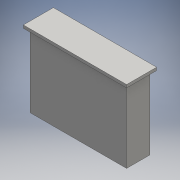
# Autodesk Inventor part: 240531_3Dstorage2
Saved by Autodesk Inventor 2016 (Build 200138000, 138)
## iProperties
Created: 2024-05-31
Part Number: 240531_3Dstorage2
Material: 일반
Document SubType Name: Modeling
Designer: pc
Density: 1 g/cm^3
Appearance: 기본값
Author: pc
Autodesk Inventor part; units mm, degrees
ref_plane "YZ Plane" through (0, 0, 0) normal (1, 0, 0) x (0, 1, 0)
ref_plane "XZ Plane" through (0, 0, 0) normal (0, 1, 0) x (-1, 0, 0)
ref_plane "XY Plane" through (0, 0, 0) normal (0, 0, 1) x (1, 0, 0)
sketch "스케치1" plane through (0, 0, 0) normal (0, 0, 1) x (1, 0, 0)
  line L0 (250, -60) -> (-250, -60)
  line L1 (-250, -60) -> (-250, 60)
  line L2 (-250, 60) -> (250, 60)
  line L3 (250, 60) -> (250, -60)
  line L4 (250, -60) -> (-250, 60) construction
  line L5 (-250, -60) -> (250, 60) construction
  point P0 (0, 0)
  dimension "d0" = 500
  dimension "d1" = 120
  constraints: 12 end point, 2 midpoint, 2 parallel, 1 horizontal, 1 perpendicular
  measures "d0" distance of L1.end L2.end
  measures "d1" distance of L2.end L0.start
extrude "돌출1" add sketch "스케치1" along normal blind 380
sketch "스케치2" plane through (0, 0, 380) normal (0, 0, 1) x (1, 0, 0)
  line L0 (-268, 78) -> (268, 78)
  line L1 (268, 78) -> (268, -78)
  line L2 (268, -78) -> (-268, -78)
  line L3 (-268, -78) -> (-268, 78)
  line L4 (250, 60) -> (-250, 60) construction
  line L5 (-250, -60) -> (250, -60) construction
  line L6 (-250, 60) -> (-250, -60) construction
  line L7 (250, -60) -> (250, 60) construction
  point P0 (0, 0)
  dimension "d4" = 18
  dimension "d5" = 18
  dimension "d6" = 18
  dimension "d7" = 18
  constraints: 8 end point, 2 parallel, 1 horizontal, 1 perpendicular
  measures "d4" distance between parallel lines of L4 L0
  measures "d5" distance between parallel lines of L2 L5
  measures "d6" distance between parallel lines of L6 L3
  measures "d7" distance between parallel lines of L1 L7
extrude "돌출2" add sketch "스케치2" along normal blind 15
shell "쉘1" thickness 15 removed faces 1 at (-83.3333, 60, 126.6667)
